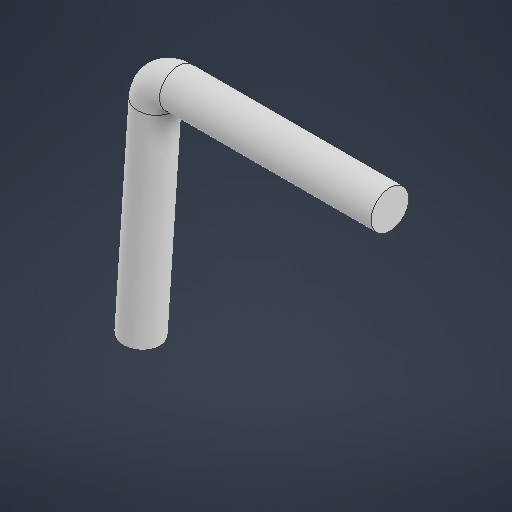
# Autodesk Inventor part: new part 3 6767
Saved by Autodesk Inventor 2026.2 (Build 302298010, 298A)
## iProperties
Created: 2026-03-16
Part Number: new part 3 6767
Material: Generic
Document SubType Name: Modeling
Designer: kerel
Density: 1 g/cm^3
Appearance: Default
Author: kerel
Autodesk Inventor part; units mm, degrees
ref_plane "YZ Plane" through (0, 0, 0) normal (1, 0, 0) x (0, 1, 0)
ref_plane "XZ Plane" through (0, 0, 0) normal (0, 1, 0) x (-1, 0, 0)
ref_plane "Work Plane1" through (-5.2551, 0.1242, 49.7367) normal (0.0698, 0.9976, 0.0024) x (-0.9976, 0.0698, 0)
sketch "Sketch1" plane through (-5.2551, 0.1242, 49.7367) normal (0.0698, 0.9976, 0.0024) x (-0.9976, 0.0698, 0)
  circle A0 centre (0, 0) radius 4.05
  point P0 (-5.251, -49.7371)
  dimension "d4" = 8.1
  constraints: 1 centre point
  measures "d4" diameter of A0
sketch3d "3D Sketch1"
  line L0 (-5.2551, 0.1242, 49.7367) -> (-2.0925, 45.3511, 49.8452)
  arc A0 (-2.0925, 45.3511, 49.8452) -> (2.8953, 50.0023, 49.8564) centre (2.8953, 45.0023, 49.8444) ccw
  line L1 (2.8953, 50.0023, 49.8564) -> (48.2327, 50.0023, 49.8564)
  dimension "d0" = 50
  dimension "d1" = 50
  dimension "d2" = 5
  dimension "d3" = 94
sweep "Sweep1" add profiles "Sketch1" path "3D Sketch1"
body "Solid1"
